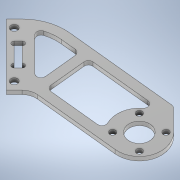
# Autodesk Inventor part: Shoulder_side_frame_
Saved by Autodesk Inventor 2020.4 (Build 244396000, 396)
## iProperties
Created: 2022-01-10
Part Number: Shoulder_side_frame_
Material: アルミニウム 2014-T4
Document SubType Name: Modeling
Designer: Masato Kubotera
Density: 2.8 g/cm^3
Appearance: 滑らか - 淡い灰色
Author: Masato Kubotera
Autodesk Inventor part; units mm, degrees
ref_plane "YZ Plane" through (0, 0, 0) normal (1, 0, 0) x (0, 1, 0)
ref_plane "XZ Plane" through (0, 0, 0) normal (0, 1, 0) x (-1, 0, 0)
ref_plane "XY Plane" through (0, 0, 0) normal (0, 0, 1) x (1, 0, 0)
sketch "スケッチ1" plane through (0, 0, 0) normal (1, 0, 0) x (0, 1, 0)
  line L0 (0, 16) -> (0, -16)
  line L1 (0, 0) -> (5, 0) construction
  line L2 (2.5, 6) -> (5, 6) construction
  line L3 (5, 6) -> (5, -6) construction
  line L4 (5, -6) -> (2.5, -6) construction
  line L5 (2.5, -6) -> (2.5, 6) construction
  line L6 (2.5, 6) -> (5, -6) construction
  line L7 (5, 6) -> (2.5, -6) construction
  circle A0 centre (2.5, 12) radius 1.6
  line L8 (2.5, 16) -> (2.5, -16) construction
  line L9 (0, 16) -> (5, 16)
  circle A1 centre (42.3, -35) radius 5.05
  line L10 (42.3, -26.5) -> (42.3, -43.5) construction
  circle A2 centre (42.3, -26.5) radius 1.35
  arc A3 (34.5925, -42.7075) -> (53.2, -35) centre (42.3, -35) ccw
  line L11 (2.45, 6.05) -> (5.05, 6.05)
  line L12 (5.05, 6.05) -> (5.05, -6.05)
  line L13 (5.05, -6.05) -> (2.45, -6.05)
  line L14 (2.45, -6.05) -> (2.45, 6.05)
  line L15 (2.45, 6.05) -> (5.05, -6.05) construction
  line L16 (5.05, 6.05) -> (2.45, -6.05) construction
  arc A4 (5.05, 3.95) -> (5.05, 6.05) centre (5.05, 5) ccw
  line L17 (3.75, 6) -> (3.75, -6) construction
  arc A5 (2.45, 6.05) -> (2.45, 3.95) centre (2.45, 5) ccw
  arc A6 (5.05, -6.05) -> (5.05, -3.95) centre (5.05, -5) ccw
  arc A7 (2.45, -3.95) -> (2.45, -6.05) centre (2.45, -5) ccw
  circle A8 centre (2.5, -12) radius 1.6
  line L18 (0, -16) -> (5, -16)
  line L19 (20.2401, 9.6874) -> (53.2, -23.2726)
  line L20 (53.2, -23.2726) -> (53.2, -35)
  line L21 (9.9251, -18.0401) -> (34.5925, -42.7075)
  circle A9 centre (33.8, -35) radius 1.35
  circle A10 centre (42.3, -43.5) radius 1.35
  circle A11 centre (50.8, -35) radius 1.35
  circle A12 centre (42.3, -35) radius 16 construction
  arc A13 (9.9251, -18.0401) -> (5, -16) centre (5, -22.9652) ccw
  line L22 (5, -16) -> (5.05, -16)
  arc A14 (20.2401, 9.6874) -> (5, 16) centre (5, -5.5527) ccw
  line L23 (9, 11.5382) -> (9, -12.7556)
  arc A15 (17.4116, 6.8589) -> (9, 11.5382) centre (5, -5.5527) ccw
  line L24 (9.3908, -12.9175) -> (23.2894, 0.9811)
  line L25 (26.1179, -1.8473) -> (12.7536, -15.2116)
  line L26 (12.7536, -15.2116) -> (31.4544, -33.9125)
  line L27 (26.1179, -1.8473) -> (49.2, -24.9294)
  arc A16 (49.2, -26.562) -> (31.4544, -33.9125) centre (42.3, -35) ccw
  line L28 (49.2, -24.9294) -> (49.2, -26.562)
  line L29 (17.4116, 6.8589) -> (23.2894, 0.9811)
  arc A17 (9.3908, -12.9175) -> (9, -12.7556) centre (5, -22.9652) ccw
  circle A18 centre (42.3, -43.5) radius 2.4 construction
  circle A19 centre (42.3, -26.5) radius 2.4 construction
  point P0 (3.75, 0)
  point P1 (2.5, 0)
  point P2 (5.05, -3.95)
  point P3 (2.45, -3.95)
  point P4 (2.45, 3.95)
  dimension "d0" = 5
  dimension "d1" = 32
  dimension "d2" = 2.5
  dimension "d3" = 12
  dimension "d4" = 3.2
  dimension "d5" = 5
  dimension "d6" = 10.1
  dimension "d7" = 17
  dimension "d8" = 2.7
  dimension "d10" = 42.3
  dimension "d11" = 1.05
  dimension "d12" = 0.05
  dimension "d13" = 0.05
  dimension "d14" = 24
  dimension "d15" = 35
  dimension "d19" = 360
  dimension "d23" = 32
  dimension "d24" = 45
  dimension "d26" = 4
  dimension "d28" = 4
  dimension "d29" = 4
  dimension "d31" = 4
  dimension "d32" = 4
  dimension "d33" = 4
  dimension "d36" = 4.8
  dimension "d37" = 4.8
  constraints: 60 end point, 20 centre point, 20 point on circle, 11 midpoint, 10 tangent, 8 symmetric about line, 7 coincident, 7 parallel, 6 point on line, 5 horizontal, 5 vertical, 4 perpendicular, 2 concentric, 1 collinear, 13 other
  measures "d0" distance of L1.end L1.start
  measures "d1" distance of L0.start L0.end
  measures "d2" distance of L3.end L4.end
  measures "d3" distance of L2.end L3.end
  measures "d4" diameter of A0
  measures "d5" distance of L0.start L9.end
  measures "d6" diameter of A1
  measures "d7" distance of L10.start L10.end
  measures "d8" diameter of A2
  measures "d10" horizontal distance of A1.centre L0.end
  measures "d11" radius of A4
  measures "d12" distance between parallel lines of L2 L11
  measures "d13" distance between parallel lines of L3 L12
  measures "d14" distance of A8.centre A0.centre
  measures "d15" vertical distance of A1.centre L1.start
  measures "d23" diameter of A12
  measures "d24" angle of L0 L19
  measures "d26" radial gap between concentric circles of A15 A14
  measures "d28" distance between parallel lines of L24 L25
  measures "d29" distance between parallel lines of L21 L26
  measures "d31" distance between parallel lines of L20 L28
  measures "d32" distance between parallel lines of L23 L3
  measures "d33" radial gap between concentric circles of A13 A17
  measures "d36" diameter of A18
  measures "d37" diameter of A19
extrude "押し出し1" add sketch "スケッチ1" along normal blind 2
fillet "フィレット1" radius 2 9 edges at (1, 9, 11.5382) (1, 9, -12.7556) (1, 9.3908, -12.9175) (1, 23.2894, 0.9811) (1, 26.1179, -1.8473) (1, 12.7536, -15.2116) (1, 31.4544, -33.9125) (1, 49.2, -26.562) (1, 49.2, -24.9294)
fillet "フィレット2" radius 2 1 edges at (1, 53.2, -23.2726)
equation "\"d13\" = d12"
